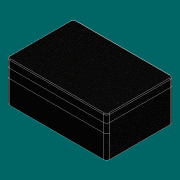
# Autodesk Inventor part: Pelican case
Saved by Autodesk Inventor 2017 (Build 210142000, 142)
## iProperties
Created: 2018-01-23
Part Number: Pelican case
Material: ABS Plastic
Document SubType Name: Modeling
Designer: Graeme_Van_Dongen
Density: 1.06 g/cm^3
Appearance: Black
Author: Graeme_Van_Dongen
Autodesk Inventor part; units mm, degrees
ref_plane "YZ Plane" through (0, 0, 0) normal (1, 0, 0) x (0, 1, 0)
sketch "Sketch1" plane through (0, 0, 0) normal (0, 1, 0) x (-1, 0, 0)
  line L0 (387.35, 258.7625) -> (-387.35, 258.7625)
  line L1 (-387.35, 258.7625) -> (-387.35, -258.7625)
  line L2 (-387.35, -258.7625) -> (387.35, -258.7625)
  line L3 (387.35, -258.7625) -> (387.35, 258.7625)
  line L4 (387.35, 258.7625) -> (-387.35, -258.7625) construction
  line L5 (-387.35, 258.7625) -> (387.35, -258.7625) construction
  point P0 (0, 0)
  dimension "d0" = 774.7
  dimension "d1" = 517.525
  constraints: 12 end point, 2 midpoint, 2 parallel, 1 horizontal, 1 perpendicular
  measures "d0" distance of L2.end L1.end
  measures "d1" distance of L1.end L0.end
extrude "Extrusion1" add sketch "Sketch1" along normal blind 307.975
ref_plane "Work Plane1" through (0, 247.65, 0) normal (0, 1, 0) x (-1, 0, 0)
split_face "Split1"
ref_plane "Work Plane2" through (0, 177.8, 0) normal (0, 1, 0) x (-1, 0, 0)
split_face "Split2"
fillet "Fillet1" radius 25.4 4 edges at (-387.35, 153.9875, 258.7625) (387.35, 153.9875, 258.7625) (387.35, 153.9875, -258.7625) (-387.35, 153.9875, -258.7625)
fillet "Fillet2" radius 6.35 8 edges at (-379.9105, 307.975, -251.323) (-379.9105, 307.975, 251.323) (379.9105, 307.975, -251.323) (379.9105, 307.975, 251.323) (387.35, 307.975, 0) (0, 307.975, -258.7625) (-387.35, 307.975, 0) (0, 307.975, 258.7625)
body "Solid1"
